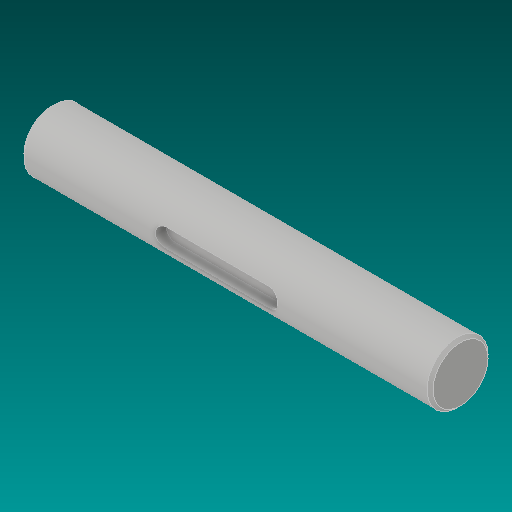
# Autodesk Inventor part: NSFMKR10-67-KA22-A20_s
Saved by Autodesk Inventor 2020 (Build 240168000, 168)
## iProperties
Created: 2022-11-16
Part Number: NSFMKR10-67-KA22-A20_s
Material: Generic
Catalog Web Link: www.cadenas.de
Description: NSFMKR, SFMKR, PSFMKR, SSFMKR, NSFHKR, SFHKR, PSFHKR, SSFHKR, NSFGKR, SFGKR, PSFGKR, SSFGKR_shafts-Rotary Shafts - Straight with Keyway -
Vendor: MISUMI
Document SubType Name: Modeling
Designer: psAdmin
Manufacturer: MISUMI
Mass: 5.15435 g
Surface Area: 23.1132 cm^2
Volume: 5.15435 cm^3
Density: 1 g/cm^3
Appearance: PSOLRGB-175-175-175
Category: PARTsolutions
Company: MISUMI
PSOL_IDENT_0: {$CADENAS_DATA/23d-libs/misumi/metric/11_rotary_shafts/11_components/psfgkr/psfgkr.prj},483 {VTYP=3D
PSOL_IDENT_1: },{NB=NSFMKR10-67-KA22-A20_s},{LINA=NSFMKR10-67-KA22-A20},{NN=NSFMKR, SFMKR, PSFMKR, SSFMKR, NSFHKR,
PSOL_IDENT_2: SFHKR, PSFHKR, SSFHKR, NSFGKR, SFGKR, PSFGKR, SSFGKR_shafts},{DATE=25.01.2022 23:09:52},{GEOMDATE=0
PSOL_IDENT_3: 5.02.2021 07:57:16},{VERSION=},{LINEID=30},{WBVAR=TS,MAT,ST,ALT1,L,NOK,KA,A,KB,B,KC,C,ALT3,FC,GALT3,
PSOL_IDENT_4: WFC,J,WALT3,V,ALT4,SFC,SGALT4,AG,ALT10,KWC,ALT11,WC,ALT6,TA,TB,ALT5,UC,ALT7,SC,ALT32,CD},{WBNUMERIC=
PSOL_IDENT_5: L,KA,A,KB,B,KC,C,FC,GALT3,WFC,J,WALT3,V,SFC,SGALT4,AG,KWC,WC,TA,TB,UC,SC}  {NB=NSFMKR10-67-KA22-A20_
PSOL_IDENT_6: s},{LINA=NSFMKR10-67-KA22-A20},{KT=DUMMY},{PN=NSFMKR10-67-KA22-A20},{TS=M},{TSALG= 'M','h9 (Cold-dra
PSOL_IDENT_7: wn)','H','h7 (Ground)','G','g6 (Ground)' },{MAT=S45C},{MATALG= 'S45C','S45C Equivalent', 'SUS304','S
PSOL_IDENT_8: US304' },{ST=},{STALG= '','-','BO','Black Oxide', 'ENP','Electroless Nickel Plating' },{TYPE=NSFMKR}
PSOL_IDENT_9: ,{D=10},{ALT1=},{L=67.0},{LALG=[15:800/0.1]},{LMIN=15},{LMAX=800},{NOK=1},{NOKALG= '1', 'with 1 Key
PSOL_IDENT_10: Groove', '2'  , 'with 2 Key Grooves', '3'  , 'with 3 Key Grooves'},{BB=3},{TT=1.8},{KA=22.0},{KAALG=
PSOL_IDENT_11: [0:64/0.1]},{KAMIN=0},{KAMAX1=64},{KAMAX2=59},{KAMAX3=54},{A=20.0},{AALG=[3:45/0.1]},{AMIN=3},{AMAX1=
PSOL_IDENT_12: 45},{AMAX2=40},{AMAX3=35},{KAPN=-KA22-A20},{KB=0.0},{KBALG=[0]},{KBMIN=44},{KBMAX1=64},{KBMAX2=59},{
PSOL_IDENT_13: B=0.0},{BALG=[0]},{BMIN=3},{BMAX1=67},{BMAX2=62},{KBPN=},{KC=0.0},{KCALG=[0]},{KCMIN=2},{KCMAX=64},{
PSOL_IDENT_14: C=0.0},{CALG=[0]},{CMIN=3},{CMAX=67},{KCPN=},{CIFKA=5},{CIFKB=3},{CIFKC=3},{ALT3=},{ALT3ALG= '', 'w/
PSOL_IDENT_15: o Set Screw Flat','FC','with FC (Adds a Set Screw Flat)','WFC','with WFC (Adds Two Set Screw Flats)'
PSOL_IDENT_16: ,'FCWFC','with FC + WFC (Adds Three Set Screw Flats)' },{ALT3PN=},{FC=0},{FCALG=[0]},{FCMIN=0},{FCMA
PSOL_IDENT_17: X=66},{GALT3=0},{GALT3ALG=[0]},{GALT3MIN=1},{GALT3MAX=67},{GALT3MAX2=61},{GALT3MAX3=64},{WFC=0},{WFC
PSOL_IDENT_18: ALG=[0]},{WFCMIN=0},{WFCMIN2=2},{WFCMAX=63},{WFCMAX2=-3},{WFCMAX3=-4},{J=0},{JALG=[0]},{JMIN=1},{JMA
PSOL_IDENT_19: X=64},{JMAX2=-2},{JMAX3=-5},{WALT3=0},{WALT3ALG=[0]},{WALT3MIN=0},{WALT3MIN2=69},{WALT3MAX=64},{WALT
PSOL_IDENT_20: 3MAX2=64},{V=0},{VALG=[0]},{VMIN=1},{VMAX=65},{VMAX3=65},{CIFFC=0},{ALT4=},{ALT4ALG= '', 'w/o SFC (2
PSOL_IDENT_21: Set Screw Flats (Angle Specified))', 'SFC' , 'with SFC (2 Set Screw Flats (Angle Specified))'},{ALT
PSOL_IDENT_22: 4PN=},{SFC=0},{SFCALG=[0]},{SFCMIN=0},{SFCMAX=66},{SGALT4=0},{SGALT4ALG=[0]},{SGALT4MIN=1},{SGALT4MA
PSOL_IDENT_23: X=50},{AG=0},{AGALG=[0]},{H=0},{CIFSFC=0},{ALT10=},{ALT10ALG= '', 'w/o KWC (2 Set Screw Flats at bot
PSOL_IDENT_24: h ends)', 'KWC', 'with KWC (2 Set Screw Flats at both ends)' },{ALT10PN=},{KWC=0},{KWCALG=[0]},{KWCM
PSOL_IDENT_25: IN=1},{KWCMAX=32.5},{WALT10=8},{ALT11=},{ALT11ALG= '','Not applicable' },{ALT11PN=},{WC=0.0},{WCALG=
PSOL_IDENT_26: [0]},{ALT6=},{ALT6ALG= '','w/o Retaining Ring Groove','TA','with TA (Retaining Ring Groove)','TB','w
PSOL_IDENT_27: ith TB (Retaining Ring Groove)','TATB','with TA + TB (Two Retaining Ring Grooves)' },{ALT6PN=},{TA=0
PSOL_IDENT_28: .0},{TAALG=[0]},{TAMIN=2},{TAMAX=0},{TB=0.0},{TBALG=[0]},{TBMIN=2},{TBMAX=0},{DDALT6=0.0},{MM=0.00},
PSOL_IDENT_29: {ALT5=},{ALT5ALG= '', 'w/o UC (Slit Cam Groove)', 'UC', 'with UC (Slit Cam Groove)'},{ALT5PN=},{UC=0
PSOL_IDENT_30: },{UCALG=[0]},{UCMIN=1},{UCMAX=61},{DD=0},{LL1=0},{ALT7=},{ALT7ALG= '', 'w/o SC (Wrench Flats)', 'SC'
PSOL_IDENT_31: , 'with SC (Wrench Flats)'},{ALT7PN=},{SC=0},{SCALG=[0]},{SCMIN=0},{SCMAX=59},{WALT7=0},{LL2=0},{LL2
PSOL_IDENT_32: ALG=8},{CIFSC=0},{ALT32=},{ALT32ALG=  '','w/o CD (Changes Part D Chamfering)','CD', 'with CD (Change
PSOL_IDENT_33: s Part D Chamfering)' },{ALT32PN=},{CD=},{CDALG= '','' },{CD3D=0.5},{CIF32=0},{CIF320=0},{CIF32FC=0}
PSOL_IDENT_34: ,{CIF32WFC=0},{CIF32WALT3=0},{ERRORPN=},{ERRORKGALT3=OK},{ERRORKGALT4=OK},{ERRORKGALT5=OK},{ERRORKGA
PSOL_IDENT_35: LT7=OK},{ERRORKGALT10=OK},{ERRORALT34=OK},{ERRORALT35=OK},{ERRORALT37=OK},{ERRORALT310=OK},{ERRORALT
PSOL_IDENT_36: 45=OK},{ERRORALT47=OK},{ERRORALT410=OK},{ERRORALT57=OK},{ERRORALT510=OK},{ERRORALT710=OK},{ERRORALT3
PSOL_IDENT_37: 6=OK},{ERRORALT46=OK},{ERRORALT56=OK},{ERRORALT67=OK},{ERRORALT610=OK},{ERRORKGALT6=OK},{CIFTA=0},{C
PSOL_IDENT_38: IFTB=0}
NB: NSFMKR10-67-KA22-A20_s
NN: NSFMKR, SFMKR, PSFMKR, SSFMKR, NSFHKR, SFHKR, PSFHKR, SSFHKR, NSFGKR, SFGKR, PSFGKR, SSFGKR_shafts
NT: Rotary Shafts - Straight with Keyway -
NBSYN: $PN._s
LINA: NSFMKR10-67-KA22-A20
CATALOG: Misumi
PN: NSFMKR10-67-KA22-A20
TS: h9 (Cold-drawn)
MAT: S45C Equivalent
ST: -
D: 10
ALT1: w/o LKC (Changes L Tolerance)
L: 67
NOK: with 1 Key Groove
KA: 22
A: 20
KB: 0
B: 0
KC: 0
C: 0
ALT3: w/o Set Screw Flat
FC: 0
GALT3: 0
WFC: 0
J: 0
WALT3: 0
V: 0
ALT4: w/o SFC (2 Set Screw Flats (Angle Specified))
SFC: 0
SGALT4: 0
AG: 0
H: 0
ALT10: w/o KWC (2 Set Screw Flats at both ends)
KWC: 0
ALT11: Not applicable
WC: 0
ALT6: w/o Retaining Ring Groove
TA: 0
TB: 0
DDALT6: 0
MM: 0
ALT5: w/o UC (Slit Cam Groove)
UC: 0
LL1: 0
ALT7: w/o SC (Wrench Flats)
SC: 0
WALT7: 0
LL2: 0
ALT32: w/o CD (Changes Part D Chamfering)
SUPPLIER: MISUMI
ARTICLENO: NSFMKR10-67-KA22-A20_s
BOMINFO: NSFMKR10-67-KA22-A20
CREATOR: CADENAS GmbH
Title: NSFMKR10-67-KA22-A20
Author: Cadenas PARTsolutions
Comments: Rotary Shafts - Straight with Keyway -
Autodesk Inventor part; units mm, degrees
ref_plane "YZ Plane" through (0, 0, 0) normal (1, 0, 0) x (0, 1, 0)
ref_plane "XZ Plane" through (0, 0, 0) normal (0, 1, 0) x (-1, 0, 0)
ref_plane "XY Plane" through (0, 0, 0) normal (0, 0, 1) x (1, 0, 0)
sketch "Sketch_1" plane through (0, 0, 0) normal (0, 1, 0) x (-1, 0, 0)
  line L0 (-67, 0) -> (0, 0)
  line L1 (0, 0) -> (0, -4.5)
  line L2 (0, -4.5) -> (-0.5, -5)
  line L3 (-0.5, -5) -> (-66.5, -5)
  line L4 (-66.5, -5) -> (-67, -4.5)
  line L5 (-67, -4.5) -> (-67, 0)
  line L6 (-67, 0) -> (0, 0)
  constraints: 14 end point
revolve "Revolution1" add sketch "Sketch_1" angle 360 about axis through (67, 0, 0) along (1, 0, 0)
sketch "_____13" plane through (0, 0, 5) normal (0, 0, 1) x (1, 0, 0)
  arc A0 (23.5, 1.5) -> (23.5, -1.5) centre (23.5, 0) ccw
  line L0 (23.5, -1.5) -> (40.5, -1.5)
  arc A1 (40.5, -1.5) -> (40.5, 1.5) centre (40.5, 0) ccw
  line L1 (40.5, 1.5) -> (23.5, 1.5)
  constraints: 4 end point, 4 point on circle, 2 centre point
extrude "Extrusion1" cut sketch "_____13" against normal blind 1.8
body "Solid1"
